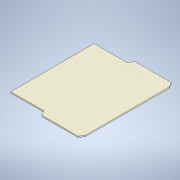
# Autodesk Inventor part: PlayerLeaderslMats_All
Saved by Autodesk Inventor 2021 (Build 250183000, 183)
## iProperties
Created: 2023-03-16
Part Number: PlayerLeaderslMats_All
Material: Paper
Document SubType Name: Modeling
Designer: Bradley
Density: 0.93 g/cm^3
Appearance: Cardboard - Chipboard
Author: Bradley
Autodesk Inventor part; units mm, degrees
ref_plane "YZ Plane" through (0, 0, 0) normal (1, 0, 0) x (0, 1, 0)
ref_plane "XZ Plane" through (0, 0, 0) normal (0, 1, 0) x (-1, 0, 0)
ref_plane "XY Plane" through (0, 0, 0) normal (0, 0, 1) x (1, 0, 0)
sketch "Sketch1" plane through (0, 0, 0) normal (0, 1, 0) x (-1, 0, 0)
  line L0 (-37.2265, 95.5) -> (37.2265, 95.5)
  line L1 (37.2265, -95.5) -> (-37.2265, -95.5)
  line L2 (43, -85.5) -> (111, -85.5)
  line L3 (111, -85.5) -> (111, 85.5)
  line L4 (111, 85.5) -> (43, 85.5)
  line L5 (-37.2265, 95.5) -> (-43, 85.5)
  line L6 (-43, 85.5) -> (-43, -85.5)
  line L7 (-43, -85.5) -> (-37.2265, -95.5)
  line L8 (37.2265, -95.5) -> (43, -85.5)
  line L9 (37.2265, 95.5) -> (43, 85.5)
  point P0 (0, 0)
  point P1 (0, 0)
  point P2 (111, 0)
  dimension "d5" = 191
  dimension "d6" = 171
  dimension "d8" = 154
  dimension "d10" = 120
  dimension "d11" = 86
  constraints: 20 end point, 2 equal length, 2 horizontal, 2 parallel, 2 perpendicular, 1 coincident, 1 horizontal alignment, 1 midpoint, 1 point on line, 1 vertical, 3 other
  measures "d5" distance between parallel lines of L0 L1
  measures "d6" distance of L2.end L3.end
  measures "d8" distance between parallel lines of L6 L3
  measures "d10" angle of L1 L8
  measures "d11" distance from line of L6 L2.start
extrude "Extrusion1" add sketch "Sketch1" along normal mid plane 2.6
body "Solid1"
